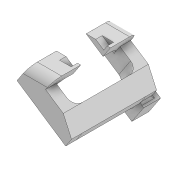
# Autodesk Inventor part: 200610 - prism holder on post for 33-69deg
Saved by Autodesk Inventor 2020.3 (Build 243373000, 373)
## iProperties
Created: 2020-06-11
Part Number: 200610 - prism holder on post for 33-69deg
Material: Generic
Document SubType Name: Modeling
Designer: Ralf
Density: 1 g/cm^3
Appearance: Default
Author: Ralf
Autodesk Inventor part; units mm, degrees
ref_plane "YZ Plane" through (0, 0, 0) normal (1, 0, 0) x (0, 1, 0)
ref_plane "XZ Plane" through (0, 0, 0) normal (0, 1, 0) x (-1, 0, 0)
ref_plane "XY Plane" through (0, 0, 0) normal (0, 0, 1) x (1, 0, 0)
sketch "Sketch1" plane through (0, 0, 0) normal (0, 0, 1) x (1, 0, 0)
  line L0 (0, 0) -> (3.7442, -2.4961)
  line L1 (0, 0) -> (4.5, 0) construction
  line L2 (3.7442, -2.4961) -> (5.4083, 0)
  line L3 (0, 0) -> (-5, 0)
  line L4 (-5, 0) -> (-6, 0)
  line L5 (-6, 0) -> (1.8981, -5.2654)
  line L6 (1.8981, -5.2654) -> (3.7442, -2.4961)
  line L7 (5.4083, 0) -> (0, 0)
  line L8 (1.8981, -5.2654) -> (-3.6489, -13.5859)
  line L9 (-6, 0) -> (-11.547, -8.3205)
  line L10 (-6, 0) -> (4, 0) construction
  line L11 (-11.547, -8.3205) -> (-3.6489, -13.5859)
  line L12 (-3.6489, -13.5859) -> (4.6716, -19.1329)
  line L13 (4.6716, -19.1329) -> (7.445, -14.9726)
  line L14 (7.445, -14.9726) -> (-0.8754, -9.4256)
  line L15 (7.445, -14.9726) -> (10.2185, -10.8123)
  line L16 (10.2185, -10.8123) -> (1.8981, -5.2654)
  line L17 (4.6716, -19.1329) -> (11.328, -23.5705)
  line L18 (11.328, -23.5705) -> (16.8747, -15.2498)
  line L19 (16.8747, -15.2498) -> (10.2185, -10.8123)
  line L20 (11.328, -23.5705) -> (14.1014, -19.4101)
  line L21 (14.1014, -19.4101) -> (10.2185, -10.8123)
  dimension "d0" = 4.5
  dimension "d1" = 33.69
  dimension "d2" = 5
  dimension "d3" = 1
  dimension "d4" = 33.69
  dimension "d5" = 10
  dimension "d6" = 10
  dimension "d7" = 123.69
  dimension "d8" = 10
  dimension "d9" = 5
  dimension "d12" = 5
  dimension "d13" = 8
  dimension "d14" = 10
  constraints: 44 end point, 5 perpendicular, 4 point on line, 3 horizontal, 2 equal length, 2 midpoint, 1 collinear, 1 parallel
  measures "d0" distance of L0.start L0.end
  measures "d1" angle of L0 L1
  measures "d2" distance of L0.start L3.end
  measures "d3" distance of L3.end L4.end
  measures "d4" angle of L5 L4
  measures "d5" distance of L5.end L8.end
  measures "d6" distance of L4.end L9.end
  measures "d7" angle of L9 L10
  measures "d8" distance of L8.end L12.end
  measures "d9" distance of L12.end L13.end
  measures "d12" distance of L13.end L15.end
  measures "d13" distance of L12.end L17.end
  measures "d14" distance of L17.end L18.end
extrude "Extrusion1" add sketch "Sketch1" along normal blind 5 contours L7 L2 L0 | L0 L6 L5 L4 L3 | L8 L11 L9 L5 | L16 L15 L14 L8 | L14 L13 L12 L8 | L21 L18 L17 L13 L15
sketch "Sketch2" plane through (0, 0, 0) normal (0, 0, -1) x (-1, 0, 0)
  line L0 (11.547, -8.3205) -> (-11.328, -23.5705) projected
  line L1 (-10.2185, -10.8123) -> (-14.1014, -19.4101)
  line L2 (-14.1014, -19.4101) -> (-11.328, -23.5705)
  line L3 (-14.1014, -19.4101) -> (-10.2185, -10.8123) projected
  line L4 (-10.2185, -10.8123) -> (-14.1014, -19.4101)
  line L5 (-14.1014, -19.4101) -> (-11.328, -23.5705)
  line L6 (-10.2185, -10.8123) -> (-1.8981, -5.2654) projected
  line L7 (11.547, -8.3205) -> (-11.328, -23.5705) projected
  line L8 (-11.328, -23.5705) -> (-14.1014, -19.4101) projected
  line L9 (-11.328, -23.5705) -> (-11.3279, -23.5704)
  line L10 (-14.1014, -19.4101) -> (-10.2185, -10.8123) projected
  line L11 (-10.2185, -10.8123) -> (-14.1014, -19.4101)
  line L12 (-14.1014, -19.4101) -> (-11.3279, -23.5704)
  line L13 (-10.2185, -10.8123) -> (-4.6715, -19.1328)
  line L14 (11.547, -8.3205) -> (-4.6716, -19.1329) projected
  line L15 (-10.2185, -10.8123) -> (-0.2185, -10.8123) construction
  line L16 (-4.6715, -19.1328) -> (-11.3279, -23.5704)
  point P0 (0, 0)
  point P1 (-4.6715, -19.1328)
  point P2 (-11.3279, -23.5704)
  dimension "d54" = 56.31
  constraints: 20 end point, 2 collinear, 2 perpendicular, 2 point on line, 1 equal length, 1 horizontal
  measures "d54" angle of L13 L15
extrude "Extrusion2" add sketch "Sketch2" along normal blind 30
sketch "Sketch3" plane through (0, 0, -30) normal (0, 0, -1) x (-1, 0, 0)
  line L0 (-11.328, -23.5705) -> (-14.1014, -19.4101) projected
  line L1 (6, 0) -> (11.547, -8.3205) projected
  line L2 (-11.328, -23.5705) -> (11.547, -8.3205)
  line L3 (11.547, -8.3205) -> (6, 0)
  line L4 (-1.8981, -5.2654) -> (-5.4083, 0) projected
  line L5 (6, 0) -> (-5.4083, 0)
  line L6 (-5.4083, 0) -> (-1.8981, -5.2654)
  line L7 (-14.1014, -19.4101) -> (-10.2185, -10.8123) projected
  line L8 (-1.8981, -5.2654) -> (-10.2185, -10.8123)
  line L9 (-10.2185, -10.8123) -> (-14.1014, -19.4101)
  line L10 (-14.1014, -19.4101) -> (-11.328, -23.5705)
  point P0 (0, 0)
  constraints: 14 end point, 3 collinear, 2 perpendicular, 1 horizontal
extrude "Extrusion3" add sketch "Sketch3" along normal blind 5
sketch "Sketch4" plane through (0, 0, -30) normal (0, 0, 1) x (1, 0, 0)
  line L0 (5.4083, 0) -> (1.8981, -5.2654) projected
  line L1 (-11.547, -8.3205) -> (-6, 0) projected
  line L2 (5.4083, 0) -> (-6, 0)
  line L3 (1.8981, -5.2654) -> (10.2185, -10.8123) projected
  line L4 (-6, 0) -> (1.8981, -5.2654)
  line L5 (1.8981, -5.2654) -> (5.4083, 0)
  point P0 (0, 0)
  point P1 (11.5682, -9.2861)
  point P2 (11.7682, -8.886)
  point P3 (10.2185, -10.8123)
  constraints: 6 end point, 1 horizontal, 1 perpendicular, 2 other
extrude "Extrusion4" add sketch "Sketch4" along normal blind 8
sketch "Sketch5" plane through (0, 0, 0) normal (0, 0, -1) x (-1, 0, 0)
  line L0 (-5.4083, 0) -> (-1.8981, -5.2654) projected
  line L1 (-5.4083, 0) -> (-1.8981, -5.2654)
  line L2 (6, 0) -> (-5.4083, 0) projected
  line L3 (-1.8981, -5.2654) -> (6, 0)
  line L4 (6, 0) -> (-5.4083, 0)
  line L5 (-5.4083, 0) -> (-1.8981, -5.2654)
  line L6 (6, 0) -> (-5.4083, 0)
  line L7 (-1.8981, -5.2654) -> (6, 0) projected
  line L8 (6, 0) -> (-1.8981, -5.2654)
  line L9 (-1.8981, -5.2654) -> (-5.4083, 0)
  point P0 (0, 0)
  constraints: 14 end point, 5 collinear, 2 perpendicular
extrude "Extrusion5" add sketch "Sketch5" along normal blind 8
fillet "Fillet1" radius 4 2 edges at (7.445, -14.9726, 0) (7.445, -14.9726, -30)
fillet "Fillet2" radius 5 2 edges at (-2.051, -2.6327, -30) (-2.051, -2.6327, 0)
sketch "Sketch6" plane through (0, 0, -22) normal (0, 0, 1) x (1, 0, 0)
  line L0 (1.8981, -5.2654) -> (5.4083, 0) projected
  line L1 (5.4083, 0) -> (3.9083, 0)
  line L2 (-6, 0) -> (5.4083, 0) projected
  line L3 (3.9083, 0) -> (2.2442, -2.4962)
  line L4 (2.2442, -2.4962) -> (-1.5, 0)
  line L5 (-1.5, 0) -> (3.9083, 0)
  point P0 (0, 0)
  point P1 (-10, 0)
  point P2 (-1.5, 0)
  dimension "d25" = 1.5
  dimension "d26" = 3
  dimension "d27" = 123.69
  dimension "d28" = 90
  constraints: 8 end point, 2 point on line, 1 collinear
  measures "d25" distance of L0.end L1.end
  measures "d26" distance of L1.end L3.end
  measures "d27" angle of L3 L1
  measures "d28" angle of L3 L4
extrude "Extrusion6" cut sketch "Sketch6" against normal blind 3
sketch "Sketch8" plane through (0, 0, -35) normal (0, 0, -1) x (-1, 0, 0)
  line L0 (-4.6716, -19.1329) -> (-11.328, -23.5705) projected
  line L1 (-11.328, -23.5705) -> (-4.6716, -19.1329)
  line L2 (-4.6716, -19.1329) -> (-0.234, -25.7893)
  line L3 (-0.234, -25.7893) -> (-6.8904, -30.2269)
  line L4 (-6.8904, -30.2269) -> (-11.328, -23.5705)
  line L5 (-11.328, -23.5705) -> (-12.9921, -24.6799)
  line L6 (-12.9921, -24.6799) -> (-7.4451, -33.0004)
  line L7 (-7.4451, -33.0004) -> (0.8754, -27.4534)
  line L8 (0.8754, -27.4534) -> (-0.234, -25.7893)
  point P0 (0, 0)
  dimension "d34" = 8
  dimension "d35" = 90
  dimension "d36" = 8
  dimension "d37" = 90
  dimension "d47" = 2
  dimension "d48" = 10
  dimension "d49" = 10
  constraints: 16 end point, 5 perpendicular, 1 collinear
  measures "d34" distance of L0.start L2.end
  measures "d35" angle of L1 L2
  measures "d36" distance of L2.end L3.end
  measures "d37" angle of L2 L3
  measures "d47" distance of L0.end L5.end
  measures "d48" distance of L5.end L6.end
  measures "d49" distance of L6.end L7.end
extrude "Extrusion8" add sketch "Sketch8" along normal blind 3 and the other way blind 5
sketch "Sketch9" plane through (0, 0, -30) normal (0, 0, 1) x (1, 0, 0)
  circle A0 centre (6.0584, -26.0666) radius 2.25
  line L0 (7.4451, -33.0004) -> (12.9921, -24.6799) projected
  line L1 (-0.8754, -27.4534) -> (7.4451, -33.0004) projected
  point P0 (0, 0)
  dimension "d44" = 4.5
  dimension "d50" = 5
  dimension "d51" = 5
  constraints: 1 centre point
  measures "d44" diameter of A0
  measures "d50" distance from line of L0 A0.centre
  measures "d51" distance from line of L1 A0.centre
extrude "Extrusion9" cut sketch "Sketch9" against normal blind 10
fillet "Fillet3" radius 1 3 edges at (4.6716, -19.1329, -32.5) (7.9998, -21.3517, -35) (11.328, -23.5705, -32.5)
fillet "Fillet4" radius 4 2 edges at (-0.2958, 0, 5) (-0.2958, 0, -35)
sketch "Sketch10" plane through (0, 0, -8) normal (0, 0, -1) x (-1, 0, 0)
  line L0 (-5.4083, 0) -> (-3.9083, 0) projected
  line L1 (-5.4083, 0) -> (-3.9083, 0)
  line L2 (-3.9083, 0) -> (-2.2442, -2.4962) projected
  line L3 (-3.9083, 0) -> (-2.2442, -2.4962)
  line L4 (-2.2442, -2.4962) -> (1.5, 0) projected
  line L5 (-2.2442, -2.4962) -> (1.5, 0)
  line L6 (1.5, 0) -> (-3.9083, 0)
  point P0 (0, 0)
  constraints: 8 end point, 4 collinear
extrude "Extrusion10" cut sketch "Sketch10" against normal blind 3
body "Solid1"
